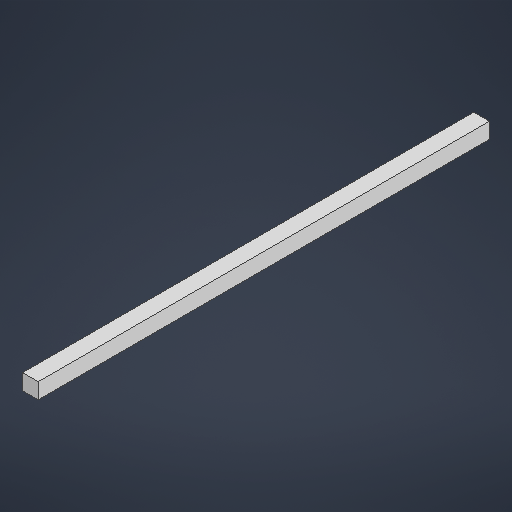
# Autodesk Inventor part: DMF 082 коллектор болванка
Saved by Autodesk Inventor 2026.2 (Build 302298000, 298)
## iProperties
Created: 2024-06-28
Part Number: DMF 082 коллектор болванка
Material: Generic
Document SubType Name: Modeling
Designer: admin
Density: 1 g/cm^3
Appearance: Default
Author: admin
Autodesk Inventor part; units mm, degrees
ref_plane "YZ Plane" through (0, 0, 0) normal (1, 0, 0) x (0, 1, 0)
ref_plane "XZ Plane" through (0, 0, 0) normal (0, 1, 0) x (-1, 0, 0)
ref_plane "XY Plane" through (0, 0, 0) normal (0, 0, 1) x (1, 0, 0)
sketch "Sketch2" plane through (0, 0, 0) normal (0, 1, 0) x (-1, 0, 0)
  line L0 (20, -490) -> (-20, -490) construction
  line L1 (-20, -490) -> (-20, 110) construction
  line L2 (-20, 110) -> (20, 110) construction
  line L3 (20, 110) -> (20, -490) construction
  line L4 (20, -490) -> (-20, 110) construction
  line L5 (-20, -490) -> (20, 110) construction
  line L6 (100, 110) -> (20, 110)
  line L7 (20, 110) -> (20, 30)
  line L8 (20, 30) -> (100, 30)
  line L9 (100, 30) -> (100, 110)
  line L10 (100, 110) -> (20, 30) construction
  line L11 (20, 110) -> (100, 30) construction
  point P0 (0, 0)
  point P1 (0, -190)
  point P2 (60, 70)
  point P3 (0, 110)
  dimension "d4" = 40
  dimension "d5" = 600
  dimension "d6" = 80
  dimension "d7" = 30
  constraints: 24 end point, 5 midpoint, 4 parallel, 3 perpendicular, 2 collinear, 2 horizontal, 1 vertical alignment
  measures "d4" distance of L1.end L2.end
  measures "d5" distance of L0.end L1.end
  measures "d6" distance of L8.end L6.start
  measures "d7" distance from line of point (0, 0) L8
extrude "Extrusion2" add sketch "Sketch2" along normal blind 2300
body "Solid2"
